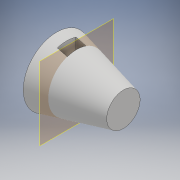
# Autodesk Inventor part: stollen_lang
Saved by Autodesk Inventor 2018 (Build 220112000, 112)
## iProperties
Created: 2018-05-14
Part Number: stollen_lang
Material: Generic
Document SubType Name: Modeling
Designer: bitbots
Density: 1 g/cm^3
Appearance: Default
Author: bitbots
Autodesk Inventor part; units mm, degrees
ref_plane "XZ Plane" through (0, 0, 0) normal (0, 1, 0) x (-1, 0, 0)
ref_plane "XY Plane" through (0, 0, 0) normal (0, 0, 1) x (1, 0, 0)
ref_plane "Work Plane1" through (6, 0, 0) normal (1, 0, 0) x (0, 1, 0)
sketch "Sketch1" plane through (0, 0, 0) normal (0, 1, 0) x (-1, 0, 0)
  line L0 (0, 0) -> (-20, 0)
  line L1 (0, 0) -> (0, -10)
  line L2 (-20, 0) -> (-20, -5)
  line L3 (-20, -5) -> (0, -10)
  dimension "d0" = 20
  dimension "d1" = 10
  dimension "d2" = 5
  constraints: 8 end point, 2 vertical, 1 horizontal
  measures "d0" distance of L0.start L0.end
  measures "d1" distance of L0.start L1.end
  measures "d2" distance of L0.end L2.end
revolve "Revolution1" add sketch "Sketch1" angle 360 about axis through (0, 0, 0) along (1, 0, 0)
sketch "Sketch2" plane through (6, 0, 0) normal (1, 0, 0) x (0, 1, 0)
  circle A0 centre (0, 0) radius 1.5
  dimension "d5" = 3
  constraints: 1 centre point, 1 coincident
  measures "d5" diameter of A0
extrude "Extrusion1" cut sketch "Sketch2" along normal blind 2 and the other way blind 10
sketch "Sketch3" plane through (6, 0, 0) normal (1, 0, 0) x (0, 1, 0)
  line L0 (0, 0) -> (2.8, 0)
  line L1 (2.8, -1.6166) -> (0, -3.2332)
  line L2 (0, -3.2332) -> (-2.8, -1.6166)
  line L3 (-2.8, -1.6166) -> (-2.8, 1.6166)
  line L4 (-2.8, 1.6166) -> (0, 3.2332)
  line L5 (0, 3.2332) -> (2.8, 1.6166)
  line L6 (2.8, 1.6166) -> (2.8, -1.6166)
  line L7 (-2.8, 1.6166) -> (2.8, 1.6166)
  line L8 (2.8, 1.6166) -> (2.8, 14.0718)
  line L9 (2.8, 14.0718) -> (-2.8, 14.0718)
  line L10 (-2.8, 14.0718) -> (-2.8, 1.6166)
  dimension "d15" = 2.8
  constraints: 22 end point, 2 horizontal, 2 parallel, 1 coincident, 1 midpoint, 1 perpendicular, 13 other
  measures "d15" distance of L0.start L0.end
extrude "Extrusion2" cut sketch "Sketch3" against normal blind 3
body "Solid1"
